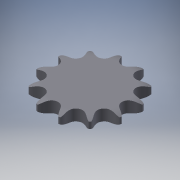
# Autodesk Inventor part: Roller Chain Sprocket1
Saved by Autodesk Inventor 2016 (Build 200138000, 138)
## iProperties
Created: 2016-05-21
Part Number: Roller Chain Sprocket1
Material: Steel
Document SubType Name: Modeling
Designer: Henrik Samuelsson
Density: 1 g/cm^3
Appearance: Steel
CustomPartVersion: 1
Author: Henrik Samuelsson
Autodesk Inventor part; units mm, degrees
ref_plane "YZ Plane" through (0, 0, 0) normal (1, 0, 0) x (0, 1, 0)
ref_plane "XZ Plane" through (0, 0, 0) normal (0, 1, 0) x (-1, 0, 0)
sketch "Theoretical Tooth Profile" plane through (0, 0, 0) normal (0, 0, 1) x (1, 0, 0)
  circle A0 centre (0, 0) radius 18.4009 construction
  line L0 (0, 0) -> (0, 18.4009) construction
  line L1 (0, 0) -> (9.2004, 15.9356) construction
  circle A1 centre (0, 0) radius 20.6314
  arc A2 (-2.4565, 16.3396) -> (2.4565, 16.3396) centre (0, 18.4009) ccw
  line L2 (0, 18.4009) -> (9.2004, 15.9356) construction
  line L3 (0, 18.4009) -> (3.8915, 21.6662) construction
  line L4 (3.8915, 21.6662) -> (-3.5138, 17.9472) construction
  arc A3 (4.9398, 20.0313) -> (3.7948, 18.5067) centre (8.5871, 16.1) ccw
  arc A4 (-3.7948, 18.5067) -> (-4.9398, 20.0313) centre (-8.5871, 16.1) ccw
  line L5 (-8.5871, 16.1) -> (-3.7948, 18.5067) construction
  arc A5 (-3.5138, 17.9472) -> (-2.4565, 16.3396) centre (3.8915, 21.6662) ccw
  line L6 (-3.5138, 17.9472) -> (-3.7948, 18.5067)
  arc A6 (2.4565, 16.3396) -> (3.5138, 17.9472) centre (-3.8915, 21.6662) ccw
  line L7 (3.7948, 18.5067) -> (3.5138, 17.9472)
  line L8 (0, 0) -> (5.3398, 19.9284) construction
  point P0 (4.6002, 17.1683)
  dimension "d0" = 36.8018
  dimension "d2" = 30
  dimension "d3" = 3.2067
  dimension "d10" = 130
  dimension "d11" = 13.333
  dimension "d12" = 5.08
  dimension "d13" = 8.2867
  dimension "d14" = 8.89
  dimension "d23" = 2.8575
  constraints: 18 end point, 15 point on circle, 7 centre point, 3 coincident, 3 point on line, 3 symmetric about line, 3 tangent, 1 equal radius, 1 midpoint, 1 parallel, 1 vertical, 1 other
  measures "d0" diameter of A0
  measures "d2" angle of L1 L0
  measures "d3" radius of A2
  measures "d10" angle of L3 L0
  measures "d11" angle of L4 L3
  measures "d12" distance of L2.start L3.end
  measures "d13" distance of L3.end L4.end
  measures "d14" distance of A3.centre L0.end
  measures "d23" distance from line of L8.end L2
sketch "Tooth Profile" plane through (0, 0, 0) normal (0, 0, 1) x (1, 0, 0)
  arc A0 (-2.9352, 17.1094) -> (2.9352, 17.1094) centre (0, 18.4009) ccw
  arc A1 (4.8622, 20.0503) -> (2.9352, 17.1094) centre (12.6997, 12.8129) ccw
  arc A2 (-2.9352, 17.1094) -> (-4.8622, 20.0503) centre (-12.6997, 12.8129) ccw
  line L0 (0, 0) -> (0, 18.4009) construction
  line L1 (0, 18.4009) -> (2.9352, 17.1094) construction
  line L2 (0, 18.4009) -> (-2.9352, 17.1094) construction
  circle A3 centre (0, 0) radius 20.6314 projected
  dimension "d44" = 132.5
  dimension "d45" = 10.668
  dimension "d46" = 3.2067
  constraints: 9 point on circle, 6 end point, 3 centre point, 2 tangent, 1 coincident, 1 equal radius, 1 vertical, 1 other
  measures "d44" angle of L2 L1
  measures "d45" radius of A1
  measures "d46" radius of A0
sketch "Section Profile" plane through (0, 0, 0) normal (1, 0, 0) x (0, 1, 0)
  line L0 (20.6314, 0) -> (-20.6314, 0) projected
  line L1 (9.2977, 2.6598) -> (-9.2977, 2.6598)
  line L2 (-9.2977, 2.6598) -> (-9.2977, -2.6598)
  line L3 (-9.2977, -2.6598) -> (9.2977, -2.6598)
  line L4 (9.2977, -2.6598) -> (9.2977, 2.6598)
  line L5 (9.2977, 2.6598) -> (20.6314, 2.6598) construction
  line L6 (20.6314, 2.6598) -> (20.6314, -2.6598) construction
  line L7 (20.6314, -2.6598) -> (9.2977, -2.6598) construction
  line L8 (9.2977, -2.6598) -> (9.2977, 2.6598)
  arc A0 (20.6314, 1.4692) -> (16.0201, 2.6598) centre (16.0201, -6.8652) ccw
  arc A1 (16.0201, -2.6598) -> (20.6314, -1.4692) centre (16.0201, 6.8652) ccw
  line L9 (16.0201, 2.6598) -> (0, 2.6598)
  line L10 (0, 2.6598) -> (0, -2.6598)
  line L11 (0, -2.6598) -> (16.0201, -2.6598)
  line L12 (0, 2.6598) -> (0, -2.6598)
  line L13 (20.6314, 1.4692) -> (20.6314, -1.4692)
  point P0 (0, 0)
  point P1 (0, 0)
  dimension "d30" = 5.3196
  dimension "d31" = 18.5954
  dimension "d32" = 5.3196
  dimension "d33" = 1.1906
  dimension "d34" = 9.525
  dimension "d43" = 2.6598
  constraints: 26 end point, 7 midpoint, 5 perpendicular, 4 parallel, 4 point on circle, 3 point on line, 3 symmetric about line, 2 centre point, 2 horizontal, 2 tangent, 1 collinear, 1 other
  measures "d30" distance between parallel lines of L7 L5
  measures "d31" distance between parallel lines of L2 L4
  measures "d32" distance between parallel lines of L3 L1
  measures "d33" distance from line of L13.start L5
  measures "d34" radius of A0
  measures "d43" distance between parallel lines of L3 L0
revolve "Shroud" add sketch "Section Profile" angle 360 about axis through (0, 0, 2.6598) along (0, 0, -1) contours L10 L3 L2 L0 | L0 L2 L1 L10
revolve "Strand" add sketch "Section Profile" angle 360 about axis through (0, 0, 2.6598) along (0, 0, -1) contours L13 A1 L11 L4 L0 | L0 L4 L9 A0 L13 | L4 L3 L10 L0 | L0 L10 L1 L4
pattern_of_one "Strand Pattern"
extrude "Theoretical Tooth" cut sketch "Theoretical Tooth Profile" along normal through all both and the other way through all contours A3 L7 A6 A2 A5 L6 A4 A1 picked at (-0.1329, 18.7826)
extrude "Tooth" [suppressed]
pattern_circular "Tooth Pattern" count 12 over 360 about axis through (0, 0, -10) along (0, 0, 1) of "Theoretical Tooth"
ref_plane "Timing Plane" through (0, 18.4009, 0) normal (1, 0, 0) x (0, 1, 0)
equation "\"d3\" = 0.5 * da_Dr + da_SC"
equation "\"d12\" = 0.8 * da_Dr"
equation "\"d13\" = 1.3 * da_Dr + da_SC"
equation "\"d14\" = 1.4 * da_Dr"
equation "\"d23\" = da_Ha"
equation "\"d44\" = da_Alfa"
equation "\"d45\" = da_Re"
equation "\"d46\" = da_Ri"
equation "\"d30\" = da_Bf"
equation "\"d31\" = da_Ds"
equation "\"d32\" = da_Bs"
equation "\"d33\" = da_Ba"
equation "\"d34\" = da_Rx"
equation "\"d40\" = da_pt"
equation "\"form_type\" = 0"
equation "\"da_p\" = 9.525"
equation "\"da_Dr\" = 6.35"
equation "\"da_SC\" = 0.03175"
equation "\"da_Ha\" = 2.8575"
equation "\"da_pt\" = 10.24"
equation "\"da_Bf\" = 5.3196"
equation "\"da_Ba\" = 1.19063"
equation "\"da_Rx\" = 9.525"
equation "\"da_Ra\" = 0.381"
equation "\"da_Bs\" = 5.3196"
equation "\"da_Ds\" = 18.59538"
equation "\"da_Re\" = 10.668"
equation "\"da_Ri\" = 3.20675"
equation "\"da_Alfa\" = 132.5deg"
body "Solid1"
